Aerotech_G74_Motor v5 (Autodesk Fusion 360 design; units mm, degrees)
Autodesk Fusion 360 part; units mm, degrees
sketch "Sketch1" plane through (0, 0, 0) normal (0, 1, 0) x (1, 0, 0)
  line L0 (-4.9075, 8.5) -> (-9.815, 0)
  line L1 (-9.815, 0) -> (-4.9075, -8.5)
  line L2 (-4.9075, -8.5) -> (4.9075, -8.5)
  line L3 (4.9075, -8.5) -> (9.815, 0)
  line L4 (9.815, 0) -> (4.9075, 8.5)
  line L5 (4.9075, 8.5) -> (-4.9075, 8.5)
  line L6 (-3.7528, -6.5) -> (3.7528, -6.5)
  line L7 (3.7528, -6.5) -> (7.5056, 0)
  line L8 (7.5056, 0) -> (3.7528, 6.5)
  line L9 (3.7528, 6.5) -> (-3.7528, 6.5)
  line L10 (-3.7528, 6.5) -> (-7.5056, 0)
  line L11 (-7.5056, 0) -> (-3.7528, -6.5)
  dimension "d1" = 17
  dimension "d4" = -2
  constraint horizontal L5
  measures "d1" distance of L2 L5
extrude "Extrude1" add sketch "Sketch1" against normal blind 11.5 makes body 1
sketch "Sketch2" plane through (0, -11.5, 0) normal (0, -1, 0) x (1, 0, 0)
  line L0 (-7.5056, 0) -> (-3.7528, 6.5)
  line L1 (-3.7528, 6.5) -> (3.7528, 6.5)
  line L2 (3.7528, 6.5) -> (7.5056, 0)
  line L3 (7.5056, 0) -> (3.7528, -6.5)
  line L4 (3.7528, -6.5) -> (-3.7528, -6.5)
  line L5 (-3.7528, -6.5) -> (-7.5056, 0)
  line L6 (-4.9075, -8.5) -> (4.9075, -8.5)
  line L7 (4.9075, -8.5) -> (9.815, 0)
  line L8 (9.815, 0) -> (4.9075, 8.5)
  line L9 (4.9075, 8.5) -> (-4.9075, 8.5)
  line L10 (-4.9075, 8.5) -> (-9.815, 0)
  line L11 (-9.815, 0) -> (-4.9075, -8.5)
  circle A0 centre (0, 0) radius 14.25
  dimension "d5" = 28.5
  constraint coincident A0.centre origin
  measures "d5" diameter of A0
extrude "Extrude2" add sketch "Sketch2" along normal blind 83.5 contours L0 L1 L2 L3 L4 L5 | L6 L7 L8 L9 L10 L11 | A0 bodies 1
sketch "Sketch3" plane through (0, -95, 0) normal (0, -1, 0) x (1, 0, 0)
  circle A0 centre (0, 0) radius 14.25
  circle A1 centre (0, 0) radius 15.85
  dimension "d8" = 31.7
  constraint coincident A0.centre A1.centre
  measures "d8" diameter of A1
extrude "Extrude3" add sketch "Sketch3" against normal blind 6.5 bodies 1
ref_plane "WorkPlane1" through (0, -99.5, 0) normal (0, -1, 0) x (1, 0, 0)
sketch "Sketch4" plane through (0, -99.5, 0) normal (0, -1, 0) x (1, 0, 0)
  circle A0 centre (0, 0) radius 7.5
  dimension "d12" = 15
  constraint coincident A0.centre origin
  measures "d12" diameter of A0
extrude "Extrude4" add sketch "Sketch4" along normal blind 13 separate body makes body 2
loft "Loft1" add section 1 face at (4.6538, -95, -3.7113) section 2 face at (0.4732, -99.5, -2.8016) on bodies 1 2 bodies 1 2
fillet "Fillet1" radius 3 6 edges at (-7.3612, -11.5, 4.25) (-7.3612, -11.5, -4.25) (0, -11.5, -8.5) (7.3612, -11.5, -4.25) (7.3612, -11.5, 4.25) (0, -11.5, 8.5) on bodies 1
